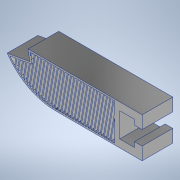
# Autodesk Inventor part: Finray_9_Kerbe_10deg
Saved by Autodesk Inventor 2022 (Build 260153000, 153)
## iProperties
Created: 2022-02-28
Part Number: Finray_9_Kerbe_10deg
Material: Generic
Document SubType Name: Modeling
Designer: richa
Density: 1 g/cm^3
Appearance: Aluminum - Flat
Author: richa
Autodesk Inventor part; units mm, degrees
ref_plane "YZ Plane" through (0, 0, 0) normal (1, 0, 0) x (0, 1, 0)
ref_plane "XZ Plane" through (0, 0, 0) normal (0, 1, 0) x (-1, 0, 0)
ref_plane "XY Plane" through (0, 0, 0) normal (0, 0, 1) x (1, 0, 0)
sketch "Sketch5" plane through (0, 0, 0) normal (0, 0, 1) x (1, 0, 0)
  line L0 (52.8, -15.6) -> (52.8, -10.6)
  line L1 (52.8, -10.6) -> (49.8, -10.6)
  line L2 (49.8, -10.6) -> (49.8, -12.6)
  line L3 (44, -12.6) -> (44, -3)
  line L4 (49.8, -3) -> (49.8, -5)
  line L5 (49.8, -5) -> (52.8, -5)
  line L6 (52.8, -5) -> (52.8, 0)
  line L7 (52.8, 0) -> (7.8, 0)
  line L8 (44, -3) -> (49.8, -3)
  line L9 (44, -12.6) -> (49.8, -12.6)
  line L10 (52.8, -15.6) -> (7.8, -15.6)
  line L11 (7.8, -15.6) -> (0, -15.6)
  line L12 (0, -15.6) -> (0, 0)
  line L13 (0, 0) -> (7.8, 0)
  point P0 (7.8, 0)
  dimension "d41" = 5.8
  dimension "d48" = 44
  dimension "d50" = 3
  dimension "d63" = 45
  dimension "d71" = 0
  dimension "d87" = 5.6
  dimension "d88" = 9.6
  dimension "d97" = 15.6
  constraints: 28 end point, 8 perpendicular, 4 collinear, 3 parallel, 2 horizontal, 1 vertical
  measures "d41" distance between parallel lines of L2 L3
  measures "d48" distance from line of L3 L12.end
  measures "d50" distance of L4.end L5.end
  measures "d63" distance of L0.start L10.end
  measures "d71" distance from line of L12.end L7
  measures "d87" distance from line of L0.end L5
  measures "d88" distance of L3.start L3.end
  measures "d97" distance of L11.end L12.end
extrude "Extrusion2" add sketch "Sketch5" along normal blind 12
sketch "Sketch8" plane through (0, 0, 0) normal (0, 0, -1) x (-1, 0, 0)
  line L0 (-8.1687, 0) -> (-8.8633, -3.9392)
  line L1 (-7.8, 0) -> (-1.143, 0) construction
  line L2 (0, -5.5021) -> (-8.8633, -3.9392)
  line L3 (-7.8, 0) -> (-8.1687, 0)
  line L4 (0, 0) -> (0, -15.6) projected
  line L5 (-52.8, 0) -> (0, 0) projected
  line L6 (-7.8, 0) -> (0, 0)
  line L7 (0, 0) -> (0, -5.5021)
  dimension "d80" = 100
  dimension "d95" = 4
  dimension "d96" = 9
  constraints: 12 end point, 2 collinear, 2 perpendicular, 1 horizontal, 1 point on line
  measures "d80" angle of L0 L1
  measures "d95" distance of L0.start L0.end
  measures "d96" distance of L2.start L0.end
extrude "Extrusion5" cut sketch "Sketch8" against normal through all
fillet "Fillet2" radius 23 1 edges at (0, -15.6, 6)
shell "Shell1" thickness 0.62 removed faces 1 at (23.9679, -7.5131, 12)
sketch "Sketch13" plane through (0, 0, 12) normal (0, 0, 1) x (1, 0, 0)
  line L0 (19.0404, -15.6) -> (52.8, -15.6) projected
  line L1 (42.0526, -15.6) -> (42.0526, 0)
  line L2 (52.8, 0) -> (8.1687, 0) projected
  line L3 (52.8, 0) -> (8.1687, 0) projected
  line L4 (52.8, -5) -> (52.8, 0) projected
  line L5 (49.8, -5) -> (52.8, -5) projected
  line L6 (49.8, -3) -> (49.8, -5) projected
  line L7 (44, -3) -> (49.8, -3) projected
  line L8 (44, -12.6) -> (44, -3) projected
  line L9 (49.8, -12.6) -> (44, -12.6) projected
  line L10 (49.8, -10.6) -> (49.8, -12.6) projected
  line L11 (52.8, -10.6) -> (49.8, -10.6) projected
  line L12 (52.8, -15.6) -> (52.8, -10.6) projected
  line L13 (42.0526, 0) -> (52.8, 0)
  line L14 (52.8, -5) -> (52.8, 0) projected
  line L15 (52.8, -5) -> (52.8, 0)
  line L16 (52.8, 0) -> (52.8, -5)
  line L17 (44, -12.6) -> (44, -3) projected
  line L18 (44, -3) -> (44, -12.6)
  line L19 (49.8, -12.6) -> (44, -12.6) projected
  line L20 (44, -12.6) -> (49.8, -12.6)
  line L21 (43.38, -13.22) -> (50.42, -13.22) projected
  line L22 (52.8, -10.6) -> (52.8, -15.6)
  line L23 (52.8, -15.6) -> (42.0526, -15.6)
  line L24 (44, -3) -> (49.8, -3) projected
  line L25 (44, -3) -> (49.8, -3)
  line L26 (49.8, -3) -> (49.8, -5)
  line L27 (49.8, -5) -> (52.8, -5)
  line L28 (52.8, -10.6) -> (49.8, -10.6)
  line L29 (49.8, -10.6) -> (49.8, -12.6)
  point P0 (0, 0)
  dimension "d102" = 10.7474
  constraints: 26 end point, 10 collinear, 2 point on line, 2 vertical, 1 parallel
  measures "d102" distance between parallel lines of L4 L1
extrude "Extrusion7" add sketch "Sketch13" against normal blind 12
sketch "Sketch14" plane through (8.9076, -0.62, 0.62) normal (0, 0, 1) x (1, 0, 0)
  line L0 (33.145, -14.36) -> (33.145, 0) projected
  line L1 (33.145, 0) -> (0, 0) projected
  line L2 (0.6739, -3.8221) -> (0, 0) projected
  line L3 (-7.835, -5.3225) -> (0.6739, -3.8221) projected
  arc A0 (-7.835, -5.3225) -> (10.1328, -14.36) centre (10.1328, 8.02) ccw projected
  line L4 (10.1328, -14.36) -> (33.145, -14.36) projected
  point P0 (-8.9076, 0.62)
extrude "Extrusion8" cut sketch "Sketch14" against normal blind 12
sketch "Sketch15" plane through (0, 0, 12) normal (0, 0, 1) x (1, 0, 0)
  line L0 (42.0526, -0.62) -> (8.9076, -0.62) construction
  line L1 (19.0404, -14.98) -> (42.0526, -14.98) projected
  line L2 (40.5378, -0.62) -> (38.0057, -14.98)
  line L3 (38.0057, -14.98) -> (37.6199, -14.98)
  line L4 (37.6199, -14.98) -> (40.1519, -0.62)
  line L5 (36.3243, -0.62) -> (36.7102, -0.62)
  line L6 (36.7102, -0.62) -> (34.0769, -15.5543)
  line L7 (34.0769, -15.5543) -> (33.691, -15.5543)
  line L8 (33.691, -15.5543) -> (36.3243, -0.62)
  line L9 (32.5026, -0.62) -> (32.8826, -0.62)
  line L10 (32.8826, -0.62) -> (30.2493, -15.5543)
  line L11 (30.2493, -15.5543) -> (29.8693, -15.5543)
  line L12 (29.8693, -15.5543) -> (32.5026, -0.62)
  line L13 (28.6672, -0.62) -> (29.0472, -0.62)
  line L14 (29.0472, -0.62) -> (26.4138, -15.5543)
  line L15 (26.4138, -15.5543) -> (26.0338, -15.5543)
  line L16 (26.0338, -15.5543) -> (28.6672, -0.62)
  line L17 (24.7984, -0.62) -> (25.1842, -0.62)
  line L18 (25.1842, -0.62) -> (22.5509, -15.5543)
  line L19 (22.5509, -15.5543) -> (22.1651, -15.5543)
  line L20 (22.1651, -15.5543) -> (24.7984, -0.62)
  line L21 (20.9296, -0.62) -> (21.3155, -0.62)
  line L22 (21.3155, -0.62) -> (18.6821, -15.5543)
  line L23 (18.6821, -15.5543) -> (18.2963, -15.5543)
  line L24 (18.2963, -15.5543) -> (20.9296, -0.62)
  line L25 (17.0608, -0.62) -> (17.4467, -0.62)
  line L26 (17.4467, -0.62) -> (14.8725, -15.2192)
  line L27 (13.2195, -0.62) -> (13.6054, -0.62)
  line L28 (13.6054, -0.62) -> (11.2065, -14.2248)
  line L29 (10.8444, -14.0901) -> (13.2195, -0.62)
  arc A0 (1.0726, -5.9425) -> (19.0404, -14.98) centre (19.0404, 7.4) ccw projected
  line L30 (42.0526, -0.62) -> (42.0526, -14.98) projected
  line L31 (1.0726, -5.9425) -> (9.5815, -4.4421) projected
  arc A1 (0, -5.5021) -> (19.0404, -15.6) centre (19.0404, 7.4) ccw projected
  line L32 (5.529, -0.62) -> (4.0181, -9.189)
  line L33 (4.3517, -9.4851) -> (5.9149, -0.62)
  line L34 (9.3703, -0.62) -> (7.4127, -11.7223)
  line L35 (7.7619, -11.9303) -> (9.7562, -0.62)
  line L36 (42.0526, -14.98) -> (19.0404, -14.98) projected
  line L37 (40.1716, -14.98) -> (40.5458, -15.046)
  line L38 (40.5458, -15.046) -> (43.0895, -0.62)
  line L39 (43.0895, -0.62) -> (42.7036, -0.62)
  line L40 (42.7036, -0.62) -> (40.1716, -14.98)
  line L41 (8.9076, -0.62) -> (42.0526, -0.62) projected
  line L42 (38.8761, -0.62) -> (39.2619, -0.62)
  line L43 (39.2619, -0.62) -> (36.7299, -14.98)
  line L44 (36.7299, -14.98) -> (36.344, -14.98)
  line L45 (36.344, -14.98) -> (38.8761, -0.62)
  line L46 (35.0485, -0.62) -> (35.4343, -0.62)
  line L47 (35.4343, -0.62) -> (32.9023, -14.98)
  line L48 (32.9023, -14.98) -> (32.5164, -14.98)
  line L49 (32.5164, -14.98) -> (35.0485, -0.62)
  line L50 (31.2267, -0.62) -> (31.6126, -0.62)
  line L51 (31.6126, -0.62) -> (29.0806, -14.98)
  line L52 (29.0806, -14.98) -> (28.6947, -14.98)
  line L53 (28.6947, -14.98) -> (31.2267, -0.62)
  line L54 (27.3776, -0.62) -> (27.7634, -0.62)
  line L55 (27.7634, -0.62) -> (25.2314, -14.98)
  line L56 (25.2314, -14.98) -> (24.8455, -14.98)
  line L57 (24.8455, -14.98) -> (27.3776, -0.62)
  line L58 (23.5088, -0.62) -> (23.8946, -0.62)
  line L59 (23.8946, -0.62) -> (21.3626, -14.98)
  line L60 (21.3626, -14.98) -> (20.9767, -14.98)
  line L61 (20.9767, -14.98) -> (23.5088, -0.62)
  line L62 (19.64, -0.62) -> (20.0259, -0.62)
  line L63 (20.0259, -0.62) -> (17.5031, -14.9271)
  line L64 (17.5031, -14.9271) -> (17.1173, -14.9271)
  line L65 (17.1173, -14.9271) -> (19.64, -0.62)
  line L66 (15.785, -0.62) -> (16.1708, -0.62)
  line L67 (16.1708, -0.62) -> (13.7506, -14.3459)
  line L68 (13.7506, -14.3459) -> (13.3647, -14.3459)
  line L69 (13.3647, -14.3459) -> (15.785, -0.62)
  line L70 (11.9299, -0.62) -> (12.3158, -0.62)
  line L71 (12.3158, -0.62) -> (10.1114, -13.1216)
  line L72 (10.1114, -13.1216) -> (9.7255, -13.1216)
  line L73 (9.7255, -13.1216) -> (11.9299, -0.62)
  line L74 (4.639, -0.62) -> (3.2557, -8.4653)
  line L75 (2.9284, -8.1328) -> (4.2532, -0.62)
  line L76 (7.7494, -4.7652) -> (7.3636, -4.7652)
  line L77 (8.0945, -0.62) -> (6.2682, -10.9775)
  line L78 (6.6126, -11.2122) -> (8.4803, -0.62)
  line L79 (41.4278, -0.62) -> (41.8136, -0.62)
  line L80 (41.8136, -0.62) -> (39.2816, -14.98)
  line L81 (39.2816, -14.98) -> (38.8957, -14.98)
  line L82 (38.8957, -14.98) -> (41.4278, -0.62)
  line L83 (37.6002, -0.62) -> (37.9861, -0.62)
  line L84 (37.9861, -0.62) -> (35.454, -14.98)
  line L85 (35.454, -14.98) -> (35.0681, -14.98)
  line L86 (35.0681, -14.98) -> (37.6002, -0.62)
  line L87 (33.7726, -0.62) -> (34.1585, -0.62)
  line L88 (34.1585, -0.62) -> (31.6264, -14.98)
  line L89 (31.6264, -14.98) -> (31.2406, -14.98)
  line L90 (31.2406, -14.98) -> (33.7726, -0.62)
  line L91 (29.9509, -0.62) -> (30.3367, -0.62)
  line L92 (30.3367, -0.62) -> (27.8047, -14.98)
  line L93 (27.8047, -14.98) -> (27.4188, -14.98)
  line L94 (27.4188, -14.98) -> (29.9509, -0.62)
  line L95 (26.088, -0.62) -> (26.4738, -0.62)
  line L96 (26.4738, -0.62) -> (23.9418, -14.98)
  line L97 (23.9418, -14.98) -> (23.5559, -14.98)
  line L98 (23.5559, -14.98) -> (26.088, -0.62)
  line L99 (22.2192, -0.62) -> (22.6051, -0.62)
  line L100 (22.6051, -0.62) -> (20.073, -14.98)
  line L101 (20.073, -14.98) -> (19.6871, -14.98)
  line L102 (19.6871, -14.98) -> (22.2192, -0.62)
  line L103 (18.3504, -0.62) -> (18.7363, -0.62)
  line L104 (18.7363, -0.62) -> (16.2353, -14.8035)
  line L105 (16.2353, -14.8035) -> (15.8495, -14.8035)
  line L106 (15.8495, -14.8035) -> (18.3504, -0.62)
  line L107 (14.4954, -0.62) -> (14.8812, -0.62)
  line L108 (14.8812, -0.62) -> (12.5204, -14.0092)
  line L109 (12.5204, -14.0092) -> (12.1345, -14.0092)
  line L110 (12.1345, -14.0092) -> (14.4954, -0.62)
  line L111 (6.4184, -4.9999) -> (6.0326, -4.9999)
  line L112 (6.8049, -0.62) -> (5.128, -10.1302)
  line L113 (5.4673, -10.3942) -> (7.1907, -0.62)
  line L114 (11.0262, -0.62) -> (10.6462, -0.62)
  line L115 (10.6462, -0.62) -> (8.4916, -12.8395)
  line L116 (8.4916, -12.8395) -> (8.8716, -12.8395)
  line L117 (8.8716, -12.8395) -> (11.0262, -0.62)
  line L118 (8.9076, -0.62) -> (-0.0004, -0.62) construction
  line L119 (40.1519, -0.62) -> (40.5378, -0.62)
  line L120 (14.607, -14.5365) -> (17.0608, -0.62)
  point P0 (0, 0)
  point P1 (5.1016, -5.2321)
  point P2 (4.716, -5.2308)
  point P3 (7.4249, -11.6533)
  point P4 (7.8105, -11.6543)
  point P5 (37.6199, -14.98)
  point P6 (33.7923, -14.98)
  point P7 (34.1781, -14.98)
  point P8 (29.9706, -14.98)
  point P9 (30.3506, -14.98)
  point P10 (26.1351, -14.98)
  point P11 (26.5151, -14.98)
  point P12 (22.2663, -14.98)
  point P13 (22.6522, -14.98)
  point P14 (19.6462, -14.98)
  point P15 (20.0321, -14.98)
  point P16 (10.9541, -13.468)
  point P17 (11.3158, -13.6047)
  point P18 (3.3866, -5.5345)
  point P19 (3.709, -5.8946)
  point P20 (3.0213, -7.6064)
  point P21 (6.4013, -10.2227)
  point P22 (6.7826, -10.2486)
  point P23 (40.1716, -14.98)
  point P24 (40.5575, -14.98)
  point P25 (36.344, -14.98)
  point P26 (36.7299, -14.98)
  point P27 (39.2619, -0.62)
  point P28 (35.0485, -0.62)
  point P29 (32.9023, -14.98)
  point P30 (35.4343, -0.62)
  point P31 (31.2267, -0.62)
  point P32 (29.0806, -14.98)
  point P33 (31.6126, -0.62)
  point P34 (27.3776, -0.62)
  point P35 (25.2314, -14.98)
  point P36 (27.7634, -0.62)
  point P37 (23.5088, -0.62)
  point P38 (21.3626, -14.98)
  point P39 (23.8946, -0.62)
  point P40 (20.0259, -0.62)
  point P41 (16.1708, -0.62)
  point P42 (12.3158, -0.62)
  point P43 (5.3359, -8.9512)
  point P44 (5.7264, -8.9245)
  point P45 (39.2816, -14.98)
  point P46 (41.8136, -0.62)
  point P47 (35.0681, -14.98)
  point P48 (35.454, -14.98)
  point P49 (37.9861, -0.62)
  point P50 (31.6264, -14.98)
  point P51 (34.1585, -0.62)
  point P52 (27.8047, -14.98)
  point P53 (30.3367, -0.62)
  point P54 (23.9418, -14.98)
  point P55 (26.4738, -0.62)
  point P56 (20.073, -14.98)
  point P57 (22.6051, -0.62)
  point P58 (18.7363, -0.62)
  point P59 (14.8812, -0.62)
  point P60 (10.6462, -0.62)
  point P61 (3.7848, -5.4643)
  point P62 (4.7034, -5.3023)
  point P63 (6.0202, -5.0701)
  point P64 (7.3512, -4.8354)
  point P65 (9.0662, -4.533)
  point P66 (8.668, -4.6032)
  point P67 (14.9801, -14.6086)
  point P68 (9.7562, -0.62)
  dimension "d105" = 0.38
  dimension "d107" = 0.38
  dimension "d108" = 0.38
  dimension "d109" = 0.38
  dimension "d110" = 0.38
  dimension "d111" = 0.38
  dimension "d113" = 0.38
  dimension "d129" = 0.38
  dimension "d131" = 0.38
  dimension "d132" = 0.38
  dimension "d133" = 0.38
  dimension "d134" = 0.38
  dimension "d135" = 0.38
  dimension "d136" = 0.38
  dimension "d137" = 0.38
  dimension "d138" = 0.38
  dimension "d139" = 0.38
  dimension "d151" = 0.38
  dimension "d157" = 0.38
  dimension "d161" = 0.38
  dimension "d163" = 0.38
  dimension "d168" = 0.89
  dimension "d169" = 0.38
  dimension "d170" = 0.89
  dimension "d171" = 0.89
  dimension "d172" = 0.38
  dimension "d173" = 0.89
  dimension "d175" = 0.38
  dimension "d176" = 0.89
  dimension "d178" = 0.38
  dimension "d179" = 0.89
  dimension "d182" = 0.89
  dimension "d184" = 0.89
  dimension "d185" = 100
  dimension "d186" = 100
  dimension "d187" = 100
  dimension "d188" = 0.89
  dimension "d189" = 0.89
  dimension "d190" = 0.89
  dimension "d191" = 0.89
  dimension "d192" = 0.89
  dimension "d193" = 0.89
  dimension "d194" = 0.89
  dimension "d195" = 0.89
  dimension "d196" = 0.89
  dimension "d197" = 0.89
  dimension "d198" = 0.89
  dimension "d200" = 0.38
  dimension "d201" = 100
  dimension "d202" = 0.89
  dimension "d203" = 0.89
  dimension "d204" = 0.89
  dimension "d205" = 0.89
  dimension "d206" = 0.89
  dimension "d207" = 0.89
  dimension "d209" = 0.89
  dimension "d210" = 0.38
  dimension "d211" = 0.38
  dimension "d212" = 0.89
  dimension "d213" = 0.89
  dimension "d214" = 0.38
  dimension "d215" = 0.38
  dimension "d216" = 0.38
  dimension "d217" = 0.89
  constraints: 228 end point, 63 parallel, 34 point on line, 27 horizontal, 3 point on circle, 1 collinear, 1 perpendicular, 60 other
  measures "d105" distance between parallel lines of L2 L4
  measures "d107" distance between parallel lines of L6 L8
  measures "d108" distance of L9.start L9.end
  measures "d109" distance of L13.start L13.end
  measures "d110" distance between parallel lines of L18 L20
  measures "d111" distance between parallel lines of L22 L24
  measures "d113" distance between parallel lines of L28 L29
  measures "d129" distance between parallel lines of L38 L40
  measures "d131" distance between parallel lines of L43 L45
  measures "d132" distance between parallel lines of L47 L49
  measures "d133" distance between parallel lines of L51 L53
  measures "d134" distance between parallel lines of L55 L57
  measures "d135" distance between parallel lines of L59 L61
  measures "d136" distance between parallel lines of L63 L65
  measures "d137" distance between parallel lines of L67 L69
  measures "d138" distance between parallel lines of L71 L73
  measures "d139" distance between parallel lines of L78 L77
  measures "d151" distance between parallel lines of L80 L82
  measures "d157" distance between parallel lines of L84 L86
  measures "d161" distance between parallel lines of L88 L90
  measures "d163" distance between parallel lines of L92 L94
  measures "d168" distance between parallel lines of L20 L59
  measures "d169" distance between parallel lines of L100 L102
  measures "d170" distance between parallel lines of L61 L100
  measures "d171" distance between parallel lines of L24 L63
  measures "d172" distance between parallel lines of L104 L106
  measures "d173" distance between parallel lines of L65 L104
  measures "d175" distance between parallel lines of L108 L110
  measures "d176" distance between parallel lines of L69 L108
  measures "d178" distance of L114.start L114.end
  measures "d179" distance between parallel lines of L73 L117
  measures "d182" distance between parallel lines of L77 L113
  measures "d184" distance between parallel lines of L29 L71
  measures "d185" angle to the sketch x axis of L38
  measures "d186" angle of L0 L43
  measures "d187" angle of L0 L2
  measures "d188" distance of L5.start L46.end
  measures "d189" distance of L46.start L87.end
  measures "d190" distance of L87.start L9.end
  measures "d191" distance of L9.start L50.end
  measures "d192" distance of L50.start L91.end
  measures "d193" distance between parallel lines of L94 L14
  measures "d194" distance between parallel lines of L16 L55
  measures "d195" distance between parallel lines of L57 L96
  measures "d196" distance between parallel lines of L98 L18
  measures "d197" distance between parallel lines of L102 L22
  measures "d198" distance of L83.start L5.end
  measures "d200" distance between parallel lines of L96 L98
  measures "d201" angle of L0 L104
  measures "d202" distance of L114.end L35.end
  measures "d203" distance of L107.start L27.end
  measures "d204" distance between parallel lines of L106 L26
  measures "d205" distance of L42.start L83.end
  measures "d206" distance of L4.end L42.end
  measures "d207" distance of L79.start L2.start
  measures "d209" distance of L39.end L79.end
  measures "d210" distance between parallel lines of L35 L34
  measures "d211" distance between parallel lines of L26 L120
  measures "d212" distance of L25.start L66.end
  measures "d213" distance of L34.start L78.end
  measures "d214" distance between parallel lines of L113 L112
  measures "d215" distance between parallel lines of L32 L33
  measures "d216" distance between parallel lines of L75 L74
  measures "d217" distance of L112.start L33.end
extrude "Extrusion9" add sketch "Sketch15" against normal blind 12 contours L102 L41 L100 L1 | A0 L24 L21 L22 | L22 L23 L24 A0 | L61 L41 L59 L1 | L64 L65 A0 | A0 L65 L41 L63 | L20 L17 L18 L1 | L105 L106 A0 | A0 L106 L41 L104 | L98 L41 L96 L1 | A0 L120 L25 L26 | L57 L41 L55 L1 | L68 L69 A0 | A0 L69 L41 L67 | A0 L29 L27 L28 | L16 L13 L14 L1 | L110 L41 L108 A0 | A0 L109 L110 | L72 L73 A0 | A0 L73 L41 L71 | L94 L41 L92 L1 | L117 L116 L115 A0 | A0 L115 L41 L117 | L53 L41 L51 L1 | A0 L34 L31 L35 | L12 L9 L10 L1 | L35 L31 L34 L41 | A0 L77 L31 L78 | L90 L41 L88 L1 | A0 L112 L31 L113 | L49 L41 L47 L1 | A0 L32 L31 L33 | L8 L5 L6 L1 | A0 L75 L31 L74 | L86 L41 L84 L1 | L45 L41 L43 L1 | L4 L41 L2 L1 | L82 L41 L80 L1 | L40 L30 L38 L1 | L40 L39 L38 L30
sketch "Sketch16" plane through (0, 0, 12) normal (0, 0, 1) x (1, 0, 0)
  arc A0 (0, -5.5021) -> (19.0404, -15.6) centre (19.0404, 7.4) ccw projected
  line L0 (9.5815, -4.4421) -> (9.3319, -3.0264) projected
  line L1 (8.1687, 0) -> (8.8242, -3.7175) projected
  line L2 (8.1687, 0) -> (8.8633, -3.9392)
  line L3 (52.8, 0) -> (8.1687, 0) projected
  line L4 (0, -5.5021) -> (8.1687, 0)
  line L5 (0, -5.5021) -> (8.8633, -3.9392)
  point P0 (0, 0)
  constraints: 6 end point, 1 collinear, 1 perpendicular
extrude "Extrusion10" cut sketch "Sketch16" against normal blind 12
equation "\"l1\" = 8"
equation "\"d1\" = 0.38"
body "Solid2"
